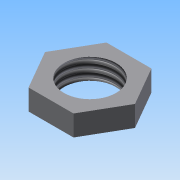
# Autodesk Inventor part: 刀轴带动盘连杆销螺帽
Saved by Autodesk Inventor 2015 (Build 190159000, 159)
## iProperties
Created: 2017-05-26
Part Number: 刀轴带动盘连杆销螺帽
Material: 常规
Document SubType Name: Modeling
Designer: Administrator
Density: 1 g/cm^3
Appearance: 默认
Author: Administrator
Autodesk Inventor part; units mm, degrees
ref_plane "YZ Plane" through (0, 0, 0) normal (1, 0, 0) x (0, 1, 0)
ref_plane "XZ Plane" through (0, 0, 0) normal (0, 1, 0) x (-1, 0, 0)
ref_plane "XY Plane" through (0, 0, 0) normal (0, 0, 1) x (1, 0, 0)
sketch "草图1" plane through (0, 0, 0) normal (0, 0, 1) x (1, 0, 0)
  circle A0 centre (0, 0) radius 5
  line L0 (4.3301, -7.5) -> (-4.3301, -7.5)
  line L1 (-4.3301, -7.5) -> (-8.6603, 0)
  line L2 (-8.6603, 0) -> (-4.3301, 7.5)
  line L3 (-4.3301, 7.5) -> (4.3301, 7.5)
  line L4 (4.3301, 7.5) -> (8.6603, 0)
  line L5 (8.6603, 0) -> (4.3301, -7.5)
  line L6 (0, 0) -> (0, 7.5)
  dimension "d0" = 10
  dimension "d1" = 15
  constraints: 14 end point, 2 coincident, 1 centre point, 1 midpoint, 1 vertical, 13 other
  measures "d0" diameter of A0
  measures "d1" distance between parallel lines of L0 L3
extrude "拉伸1" add sketch "草图1" along normal blind 4
thread "螺纹1" size "M10x1.5" class "6H" standard "ANSI Metric M Profile" full length
